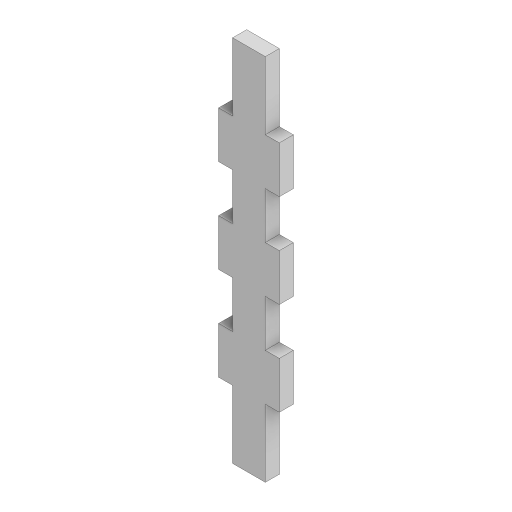
# Autodesk Inventor part: Side piece 2x
Saved by Autodesk Inventor 2023.3 (Build 273359000, 359)
## iProperties
Created: 2024-09-20
Part Number: Side piece 2x
Material: Generic
Document SubType Name: Modeling
Designer: David Zindović
Density: 1 g/cm^3
Appearance: Default
Author: David Zindović
Autodesk Inventor part; units mm, degrees
ref_plane "YZ Plane" through (0, 0, 0) normal (1, 0, 0) x (0, 1, 0)
ref_plane "XZ Plane" through (0, 0, 0) normal (0, 1, 0) x (-1, 0, 0)
ref_plane "XY Plane" through (0, 0, 0) normal (0, 0, 1) x (1, 0, 0)
sketch "Sketch1" plane through (0, 0, 0) normal (0, 0, 1) x (1, 0, 0)
  line L0 (-6.5, 39.5) -> (6.5, 39.5)
  line L1 (6.5, 39.5) -> (6.5, -39.5)
  line L2 (6.5, -39.5) -> (-6.5, -39.5)
  line L3 (-6.5, -39.5) -> (-6.5, 39.5)
  line L4 (-1.5, 39.5) -> (1.5, 39.5)
  line L5 (1.5, 39.5) -> (1.5, 36.5)
  line L6 (1.5, 36.5) -> (-1.5, 36.5)
  line L7 (-1.5, 36.5) -> (-1.5, 39.5)
  line L8 (-6.5, 5) -> (-3.5, 5)
  line L9 (-3.5, 5) -> (-3.5, -5)
  line L10 (-3.5, -5) -> (-6.5, -5)
  line L11 (-6.5, -5) -> (-6.5, 5)
  line L12 (2.5, 39.5) -> (6.5, 39.5)
  line L13 (6.5, 39.5) -> (6.5, -39.5)
  line L14 (6.5, -39.5) -> (2.5, -39.5)
  line L15 (2.5, -39.5) -> (2.5, 39.5) construction
  line L16 (2.5, 15) -> (-6.5, 15)
  line L17 (-6.5, 15) -> (-6.5, 25)
  line L18 (-6.5, 25) -> (2.5, 25)
  line L19 (2.5, 25) -> (2.5, 15)
  line L20 (0, 0) -> (2.358, 0)
  line L21 (2.5, -15) -> (-6.5, -15)
  line L22 (-6.5, -25) -> (2.5, -25)
  line L23 (0, 0) -> (0, 1.2085)
  line L24 (6.5, 5) -> (3.5, 5)
  line L25 (3.5, -5) -> (6.5, -5)
  line L26 (-2.5, 15) -> (6.5, 15)
  line L27 (6.5, 25) -> (-2.5, 25)
  line L28 (-2.5, -15) -> (6.5, -15)
  line L29 (6.5, -25) -> (-2.5, -25)
  line L30 (-3.5, -15) -> (-3.5, -25)
  line L31 (-3.5, 15) -> (-3.5, 25)
  line L32 (3.5, -5) -> (3.5, 5)
  line L33 (3.5, 15) -> (3.5, 25)
  line L34 (3.5, -25) -> (3.5, -15)
  line L35 (-3.5, 25) -> (-3.5, 39.5)
  line L36 (-3.5, 15) -> (-3.5, -39.5)
  line L37 (3.5, -39.5) -> (3.5, 39.5)
  point P0 (0, 39.5)
  point P1 (0, 36.5)
  point P2 (-3.5, 0)
  point P3 (6.5, 0)
  point P4 (-5, 5)
  point P5 (-2, 15)
  point P6 (-2, -15)
  point P7 (5, 5)
  point P8 (2, 15)
  point P9 (2, -15)
  point P10 (-6.5, -25)
  point P11 (2.5, -25)
  point P12 (6.5, -25)
  point P13 (6.5, -25)
  point P14 (6.5, -15)
  point P15 (6.5, -15)
  point P16 (6.5, -5)
  point P17 (6.5, -5)
  point P18 (6.5, 5)
  point P19 (6.5, 5)
  point P20 (6.5, 15)
  point P21 (6.5, 15)
  point P22 (6.5, 25)
  point P23 (6.5, 25)
  point P24 (2.5, 25)
  point P25 (-6.5, 15)
  point P26 (-2, 5)
  point P27 (-6.5, -5)
  point P28 (-2, -5)
  point P29 (2.5, -15)
  point P30 (-6.5, -15)
  point P31 (-3.5, -15)
  point P32 (-3.5, -25)
  point P33 (3.5, -25)
  point P34 (3.5, -15)
  point P35 (3.5, 15)
  point P36 (3.5, 25)
  dimension "d0" = 79
  dimension "d1" = 13
  dimension "d2" = 3
  dimension "d3" = 3
  dimension "d4" = 3
  dimension "d5" = 10
  dimension "d6" = 4
  dimension "d7" = 10
  dimension "d11" = 10
  constraints: 76 end point, 23 point on line, 20 symmetric about line, 10 parallel, 9 perpendicular, 6 horizontal, 6 midpoint, 2 horizontal alignment, 2 vertical, 2 vertical alignment
  measures "d0" distance of L0.end L1.end
  measures "d1" distance of L0.start L0.end
  measures "d2" distance of L4.end L5.end
  measures "d3" distance of L5.end L6.end
  measures "d4" distance of L9.end L10.end
  measures "d5" distance of L8.end L9.end
  measures "d6" distance of L13.end L14.end
  measures "d7" distance of L16.end L17.end
  measures "d11" distance between parallel lines of L16 L8
extrude "Extrusion1" add sketch "Sketch1" along normal mid plane 3 contours L0 L7 L6 L5 L37 L27 L18 L35 | L18 L31 L16 L3 | L0 L5 L6 L7 | L18 L19 L16 L31 | L16 L26 L37 L32 L28 L21 L36 L9 | L8 L9 L10 L3 | L27 L33 L26 L19 | L27 L1 L26 L33 | L21 L30 L22 L3 | L21 L28 L34 L29 L22 L30 | L24 L1 L25 L32 | L22 L29 L37 L2 L36 | L28 L1 L29 L34
equation "\"d11\" = d7"
body "Solid1"
